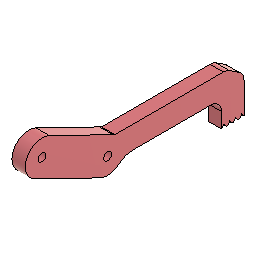
07 Pinza (Autodesk Fusion 360 design; units mm, degrees)
Autodesk Fusion 360 part; units mm, degrees
sketch "Boceto1" plane through (0, 0, 0) normal (1, 0, 0) x (0, 1, 0)
  circle A0 centre (108, 5) radius 1.75
  circle A1 centre (108, 35) radius 1.75
  circle A2 centre (76.9524, -5) radius 1.75
  circle A3 centre (76.9524, 45) radius 1.75
  circle A4 centre (44.6182, 13.9934) radius 8.1211
  circle A5 centre (24.889, 34.8767) radius 1.75
  circle A6 centre (25, 5) radius 1.75
  arc A7 (5.2265, 41.4843) -> (3, 37.3241) centre (8, 37.3241) ccw
  line L0 (3, 37.3241) -> (3, 2.6759)
  arc A8 (3, 2.6759) -> (5.2265, -1.4843) centre (8, 2.6759) ccw
  line L1 (5.2265, -1.4843) -> (31.7404, -19.1603)
  arc A9 (31.7404, -19.1603) -> (34.5139, -20) centre (34.5139, -15) ccw
  line L2 (34.5139, -20) -> (81.4861, -20)
  arc A10 (81.4861, -20) -> (84.2596, -19.1603) centre (81.4861, -15) ccw
  line L3 (84.2596, -19.1603) -> (110.7735, -1.4843)
  arc A11 (110.7735, -1.4843) -> (113, 2.6759) centre (108, 2.6759) ccw
  line L4 (113, 2.6759) -> (113, 37.3241)
  arc A12 (113, 37.3241) -> (110.7735, 41.4843) centre (108, 37.3241) ccw
  line L5 (110.7735, 41.4843) -> (84.2596, 59.1603)
  arc A13 (84.2596, 59.1603) -> (81.4861, 60) centre (81.4861, 55) ccw
  line L6 (81.4861, 60) -> (34.5139, 60)
  arc A14 (34.5139, 60) -> (31.7404, 59.1603) centre (34.5139, 55) ccw
  line L7 (31.7404, 59.1603) -> (5.2265, 41.4843)
  circle A15 centre (108, 35) radius 1.75
  line L8 (76.9524, 45) -> (108, 35) construction
  line L9 (79.2518, 52.1388) -> (110.2993, 42.1388)
  line L10 (74.6531, 37.8612) -> (105.7007, 27.8612)
  arc A16 (79.2518, 52.1388) -> (74.6531, 37.8612) centre (76.9524, 45) ccw
  arc A17 (105.7007, 27.8612) -> (109.4674, 42.355) centre (108, 35) ccw
  dimension "d1" = 15
  dimension "d2" = 15
  constraint concentric A1 A15
  constraint coincident A3.centre L8.start
  constraint coincident A1.centre A15.centre
  constraint concentric A3 A16
  constraint concentric A15 A17
  constraint parallel L8 L10
  constraint tangent L9 A16
  constraint tangent L9 A17
  constraint tangent L10 A16
  constraint coincident L5 A17.end
  constraint coincident A17 L9.end
  measures "d1" diameter of A16
  measures "d2" diameter of A17
extrude "Extruir1" add sketch "Boceto1" against normal up to surface (6 mm away) contours L4 A12 L5 L9 L10 A16 A17 | L4 A12 L5 A17
move_body "Desplazar1" bodies 1 to x (1, 0, 0) y (0, 1, 0) z (0, 0, 1) at (19.3498, 52.7891, -3.1087)
move_body "Desplazar2" bodies 1 to x (1, 0, 0) y (0, 0.965926, 0.258819) z (0, -0.258819, 0.965926) at (0, 15.2631, -32.1522)
move_body "Desplazar3" bodies 1 to x (1, 0, 0) y (0, 1, 0) z (0, 0, 1) at (-19.3498, -129.7416, -41.8913)
move_body "Desplazar4" bodies 1 to x (1, 0, 0) y (0, 0.998719, 0.050593) z (0, -0.050593, 0.998719) at (0, 0, 0)
move_body "Desplazar5" bodies 1 to x (1, 0, 0) y (0, 0.898794, -0.438371) z (0, 0.438371, 0.898794) at (0, 0, 0)
sketch "Boceto2" plane through (0, 0, 0) normal (1, 0, 0) x (0, 1, 0)
  circle A0 centre (0, 0) radius 1.75
  circle A1 centre (29.3288, -14.2749) radius 1.75
  arc A2 (3.2823, 6.7436) -> (-3.2823, -6.7436) centre (0, 0) ccw
  line L0 (-3.2823, -6.7436) -> (26.0466, -21.0185)
  arc A3 (26.0466, -21.0185) -> (31.818, -7.2) centre (29.3288, -14.2749) ccw
  line L1 (31.818, -7.2) -> (31.6834, -7.0797)
  line L2 (31.6834, -7.0797) -> (3.2823, 6.7436)
  line L3 (29.3288, -14.2749) -> (-10.6712, -14.2749) construction
  line L4 (-10.6712, -14.2749) -> (-10.6712, -44.2749) construction
  line L5 (-10.6712, -29.2749) -> (138.5011, -29.2749) construction
  line L6 (32.1886, -7.5312) -> (82.6111, -7.5312)
  line L7 (82.6111, -7.5312) -> (90.4099, -12.5927)
  line L8 (90.4099, -12.5927) -> (90.4099, -29.2749)
  line L9 (36.085, -17.5312) -> (79.6505, -17.5312)
  line L10 (79.6505, -17.5312) -> (80.4099, -18.0241)
  line L11 (80.4099, -18.0241) -> (80.4099, -29.2749)
  line L12 (80.4099, -29.2749) -> (81.3837, -27.9182)
  line L13 (81.3837, -27.9182) -> (82.4429, -29.2749)
  line L14 (83.0656, -29.2749) -> (84.0394, -27.9182)
  line L15 (84.0394, -27.9182) -> (85.0986, -29.2749)
  line L16 (85.7213, -29.2749) -> (86.695, -27.9182)
  line L17 (86.695, -27.9182) -> (87.7543, -29.2749)
  line L18 (88.3769, -29.2749) -> (89.3507, -27.9182)
  line L19 (89.3507, -27.9182) -> (90.4099, -29.2749)
  line L20 (82.4429, -29.2749) -> (83.0656, -29.2749)
  line L21 (85.0986, -29.2749) -> (85.7213, -29.2749)
  line L22 (87.7543, -29.2749) -> (88.3769, -29.2749)
  line L23 (81.3837, -27.9182) -> (81.3837, -29.2749) construction
  dimension "d8" = 40
  dimension "d10" = 30
  dimension "d15" = 7.967
  dimension "d16" = 0
  dimension "d17" = 1.3566
  constraint coincident A1.centre A3.centre
  constraint perpendicular L3 L4
  constraint midpoint L4 L5.start
  constraint perpendicular L4 L5
  constraint horizontal L6
  constraint coincident L5 L8.end
  constraint perpendicular L5 L8
  constraint coincident A3 L9.start
  constraint coincident L5 L13.end
  constraint parallel L5 L20
  constraint coincident L5 L23.end
  constraint perpendicular L5 L23
  measures "d8" distance of A1.centre L3.end
  measures "d10" distance of L3.end L4.end
  measures "d17" distance of L18.end L22
extrude "Extruir2" add sketch "Boceto2" against normal up to surface (6 mm away) contours A3 L6 L7 L8 L9 L10 L11 L12 L13 L14 L15 L16 L17 L18 L19 L20 L21 L22
fillet "Empalme1" radius 10 1 edges at (-3, 36.085, -17.5312)
fillet "Empalme2" radius 5 3 edges at (-3, 82.6111, -7.5312) (-3, 90.4099, -12.5927) (-3, 80.4099, -18.0241)
fillet "Empalme3" radius 5 1 edges at (-3, 79.6505, -17.5312)
equation "d6 = 154 deg - 180 deg"
named bodies: "Pinza"
